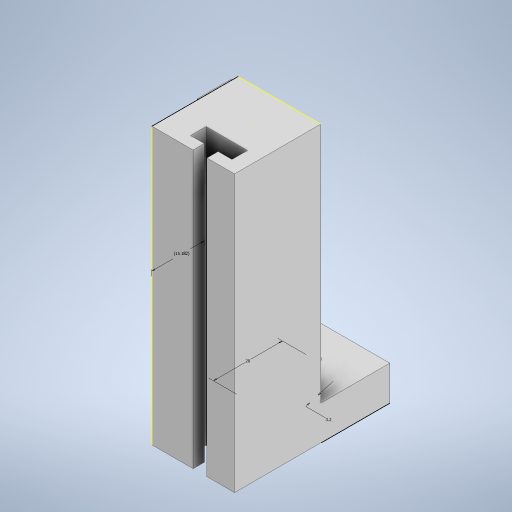
# Autodesk Inventor part: spoutstand
Saved by Autodesk Inventor 2023 (Build 270158000, 158)
## iProperties
Created: 2025-10-02
Part Number: spoutstand
Material: Generic
Document SubType Name: Modeling
Designer: ptato_qo49uko
Density: 1 g/cm^3
Appearance: Default
Author: ptato_qo49uko
Autodesk Inventor part; units mm, degrees
ref_plane "YZ Plane" through (0, 0, 0) normal (1, 0, 0) x (0, 1, 0)
ref_plane "XZ Plane" through (0, 0, 0) normal (0, 1, 0) x (-1, 0, 0)
ref_plane "XY Plane" through (0, 0, 0) normal (0, 0, 1) x (1, 0, 0)
sketch "Sketch1" plane through (0, 0, 0) normal (0, 1, 0) x (-1, 0, 0)
  line L0 (14, 15.1822) -> (-10, 15.1822)
  line L1 (-10, 15.1822) -> (-10, -9.8178)
  line L2 (-10, -9.8178) -> (14, -9.8178)
  line L3 (14, -9.8178) -> (14, 15.1822)
  point P0 (0, 0)
  dimension "d0" = 24
  dimension "d1" = 25
  constraints: 8 end point, 2 parallel, 1 horizontal, 1 perpendicular
  measures "d0" distance of L2.end L1.end
  measures "d1" distance of L1.end L0.end
extrude "Extrusion1" add sketch "Sketch1" along normal blind 80
sketch "Sketch2" plane through (0, 80, 0) normal (0, 1, 0) x (1, 0, 0)
  line L0 (-6, -11.9322) -> (-2, -11.9322)
  line L1 (-2, -11.9322) -> (-2, -15.1822)
  line L2 (2, -15.1822) -> (2, -11.9322)
  line L3 (-2, -15.1822) -> (2, -15.1822)
  line L4 (2, -11.9322) -> (6, -11.9322)
  line L5 (6, -11.9322) -> (6, -7.4322)
  line L6 (-6, -11.9322) -> (-6, -7.4322)
  line L7 (-6, -7.4322) -> (6, -7.4322)
  point P0 (0, 0)
  dimension "d8" = 4
  dimension "d118" = 3.25
  dimension "d119" = 4
  dimension "d120" = 12
  dimension "d121" = 4.5
  dimension "d122" = 4
  constraints: 16 end point, 2 horizontal, 2 vertical, 1 perpendicular, 1 point on line
  measures "d8" distance of L0.start L0.end
  measures "d118" distance of L0.end L1.end
  measures "d119" distance of L2.end L4.end
  measures "d120" distance of L6.end L5.end
  measures "d121" distance of L4.end L5.end
  measures "d122" distance of L1.end L2.start
extrude "Extrusion2" cut sketch "Sketch2" against normal blind 80
sketch "Sketch3" plane through (0, 0, 0) normal (0, -1, 0) x (1, 0, 0)
  line L0 (-14, -9.8178) -> (-14, 15.1822) projected
  line L1 (-14, -9.8178) -> (-14, -29.8178)
  line L2 (-14, -29.8178) -> (10, -29.8178)
  line L3 (10, -9.8178) -> (-14, -9.8178) projected
  line L4 (10, -29.8178) -> (10, -9.8178)
  line L5 (-14, -19.8178) -> (-2, -19.8178)
  circle A0 centre (-2, -19.8178) radius 1.6
  point P0 (0, 0)
  dimension "d121" = 4.5
  dimension "d13" = 20
  dimension "d127" = 3.2
  constraints: 8 end point, 2 perpendicular, 1 centre point, 1 coincident, 1 horizontal, 1 midpoint, 1 vertical
  measures "d13" distance of L0.start L1.end
  measures "d127" diameter of A0
extrude "Extrusion3" add sketch "Sketch3" against normal blind 10 contours A0 | L3 L4 L2 L1
sketch "Sketch4" plane through (-14, 0, 15.1822) normal (-1, 0, 0) x (0, 0, 1)
  line L0 (-25, 2.2028) -> (-15.1822, 2.2028)
  line L1 (-15.1822, 2.2028) -> (-15.1822, 1.2028)
  line L2 (-15.1822, 1.2028) -> (-25, 1.2028)
  line L3 (-25, 1.2028) -> (-25, 2.2028)
  line L4 (-25, 3.2028) -> (-25, 4.2028)
  line L5 (-25, 5.2028) -> (-25, 6.2028)
  line L6 (-25, 7.2028) -> (-25, 8.2028)
  line L7 (-25, 9.2028) -> (-25, 10.2028)
  line L8 (-25, 3.2028) -> (-25, 4.2028)
  line L9 (-25, 6.2028) -> (-15.1822, 6.2028)
  line L10 (-15.1822, 6.2028) -> (-15.1822, 5.2028)
  line L11 (-15.1822, 5.2028) -> (-25, 5.2028)
  line L12 (-25, 5.2028) -> (-25, 6.2028)
  line L13 (-25, 7.2028) -> (-25, 8.2028)
  line L14 (-25, 10.2028) -> (-15.1822, 10.2028)
  line L15 (-15.1822, 10.2028) -> (-15.1822, 9.2028)
  line L16 (-15.1822, 9.2028) -> (-25, 9.2028)
  line L17 (-25, 9.2028) -> (-25, 10.2028)
  line L18 (-25, 11.2036) -> (-25, 12.2036)
  line L19 (-25, 13.2036) -> (-25, 14.2036)
  line L20 (-25, 15.2036) -> (-25, 16.2036)
  line L21 (-25, 11.2036) -> (-25, 12.2036)
  line L22 (-25, 14.2036) -> (-15.1822, 14.2036)
  line L23 (-15.1822, 14.2036) -> (-15.1822, 13.2036)
  line L24 (-15.1822, 13.2036) -> (-25, 13.2036)
  line L25 (-25, 13.2036) -> (-25, 14.2036)
  line L26 (-25, 15.2036) -> (-25, 16.2036)
  line L27 (-15.1822, 18.2036) -> (-15.1822, 17.2036)
  line L28 (-15.1822, 22.2036) -> (-15.1822, 21.2036)
  line L29 (-25, 18.2036) -> (-15.1822, 18.2036)
  line L30 (-15.1822, 17.2036) -> (-25, 17.2036)
  line L31 (-15.1822, 21.2036) -> (-24.9999, 21.2036)
  line L32 (-24.9999, 22.2036) -> (-15.1822, 22.2036)
  line L33 (-25, 17.2036) -> (-25, 18.2036)
  line L34 (-24.9999, 19.2036) -> (-24.9999, 20.2036)
  line L35 (-25, 17.2036) -> (-25, 18.2036)
  line L36 (-24.9999, 19.2036) -> (-24.9999, 20.2036)
  line L37 (-24.9999, 21.2036) -> (-24.9999, 22.2036)
  line L38 (-24.9999, 21.2036) -> (-24.9999, 22.2036)
  line L39 (-24.9999, 23.2036) -> (-24.9999, 24.2036)
  line L40 (-24.9999, 23.2036) -> (-24.9999, 24.2036)
  line L41 (-24.9999, 24.2036) -> (-25, 25.2036)
  line L42 (-25, 10) -> (-25, 80) projected
  line L43 (-25, 25.2036) -> (-15.1821, 25.2036)
  line L44 (-15.1821, 25.2036) -> (-15.1821, 26.2036)
  line L45 (-15.1821, 26.2036) -> (-25, 26.2036)
  line L46 (-25, 26.2036) -> (-25, 25.2036)
  line L47 (-25, 26.2036) -> (-25, 27.2036)
  line L48 (-25, 28.2036) -> (-25, 27.2036)
  line L49 (-25, 28.2036) -> (-25, 29.2036)
  line L50 (-25, 29.2036) -> (-15.1821, 29.2036)
  line L51 (-15.1821, 29.2036) -> (-15.1821, 30.2036)
  line L52 (-15.1821, 30.2036) -> (-25, 30.2036)
  line L53 (-25, 30.2036) -> (-25, 29.2036)
  line L54 (-25, 30.2036) -> (-25, 31.2036)
  line L55 (-25, 32.2036) -> (-25, 31.2036)
  line L56 (-25, 32.2036) -> (-25, 33.2036)
  line L57 (-25, 33.2036) -> (-15.1821, 33.2036)
  line L58 (-15.1821, 33.2036) -> (-15.1821, 34.2036)
  line L59 (-15.1821, 34.2036) -> (-25, 34.2036)
  line L60 (-25, 34.2036) -> (-25, 33.2036)
  line L61 (-25, 34.2036) -> (-25, 35.2036)
  line L62 (-25, 36.2036) -> (-25, 35.2036)
  line L63 (-25, 36.2036) -> (-25, 37.2036)
  line L64 (-25, 37.2036) -> (-15.1821, 37.2036)
  line L65 (-15.1821, 37.2036) -> (-15.1821, 38.2036)
  line L66 (-15.1821, 38.2036) -> (-25, 38.2036)
  line L67 (-25, 38.2036) -> (-25, 37.2036)
  line L68 (-25, 40.2036) -> (-25, 39.2036)
  line L69 (-25, 40.2036) -> (-25, 41.2036)
  line L70 (-25, 41.2036) -> (-15.1822, 41.2036)
  line L71 (-15.1822, 41.2036) -> (-15.1822, 42.2036)
  line L72 (-15.1822, 42.2036) -> (-25, 42.2036)
  line L73 (-25, 42.2036) -> (-25, 41.2036)
  line L74 (-25, 42.2036) -> (-25, 43.2036)
  line L75 (-25, 44.2036) -> (-25, 43.2036)
  line L76 (-25, 44.2036) -> (-25, 45.2036)
  line L77 (-25, 45.2036) -> (-15.1822, 45.2036)
  line L78 (-15.1822, 45.2036) -> (-15.1822, 46.2036)
  line L79 (-15.1822, 46.2036) -> (-25, 46.2036)
  line L80 (-25, 46.2036) -> (-25, 45.2036)
  line L81 (-25, 46.2036) -> (-25, 47.2036)
  line L82 (-25, 48.2036) -> (-25, 47.2036)
  line L83 (-25, 48.2036) -> (-25, 49.2036)
  line L84 (-25, 49.2036) -> (-15.1822, 49.2036)
  line L85 (-15.1822, 49.2036) -> (-15.1822, 50.2036)
  line L86 (-15.1822, 50.2036) -> (-25, 50.2036)
  line L87 (-25, 50.2036) -> (-25, 49.2036)
  line L88 (-25, 50.2036) -> (-25, 51.2036)
  line L89 (-25, 52.2036) -> (-25, 51.2036)
  line L90 (-25, 38.2036) -> (-25, 39.2036)
  line L91 (-15.1821, 57.2036) -> (-15.1821, 58.2036)
  line L92 (-15.1821, 61.2036) -> (-15.1821, 62.2036)
  line L93 (-15.1821, 62.2036) -> (-25, 62.2036)
  line L94 (-25, 61.2036) -> (-15.1821, 61.2036)
  line L95 (-15.1821, 58.2036) -> (-25, 58.2036)
  line L96 (-25, 57.2036) -> (-15.1821, 57.2036)
  line L97 (-25, 53.2036) -> (-15.1821, 53.2036)
  line L98 (-15.1821, 54.2036) -> (-25, 54.2036)
  line L99 (-25, 65.2036) -> (-15.1821, 65.2036)
  line L100 (-15.1821, 66.2036) -> (-25, 66.2036)
  line L101 (-15.1821, 65.2036) -> (-15.1821, 66.2036)
  line L102 (-15.1821, 53.2036) -> (-15.1821, 54.2036)
  line L103 (-25, 54.2036) -> (-25, 53.2036)
  line L104 (-25, 54.2036) -> (-25, 55.2036)
  line L105 (-25, 56.2036) -> (-25, 55.2036)
  line L106 (-25, 56.2036) -> (-25, 57.2036)
  line L107 (-25, 58.2036) -> (-25, 57.2036)
  line L108 (-25, 58.2036) -> (-25, 59.2036)
  line L109 (-25, 66.2036) -> (-25, 65.2036)
  line L110 (-25, 64.2036) -> (-25, 65.2036)
  line L111 (-25, 64.2036) -> (-25, 63.2036)
  line L112 (-25, 62.2036) -> (-25, 63.2036)
  line L113 (-25, 60.2036) -> (-25, 61.2036)
  line L114 (-25, 60.2036) -> (-25, 59.2036)
  line L115 (-25, 62.2036) -> (-25, 61.2036)
  line L116 (-25, 52.2036) -> (-25, 53.2036)
  line L117 (-15.1812, 73.2624) -> (-15.1812, 74.2624)
  line L118 (-15.1812, 69.2624) -> (-15.1812, 70.2624)
  line L119 (-24.9991, 77.2624) -> (-15.1812, 77.2624)
  line L120 (-15.1812, 74.2624) -> (-24.9991, 74.2624)
  line L121 (-24.9991, 73.2624) -> (-15.1812, 73.2624)
  line L122 (-15.1812, 70.2624) -> (-24.9991, 70.2624)
  line L123 (-24.9991, 69.2624) -> (-15.1812, 69.2624)
  line L124 (-15.1812, 78.2624) -> (-24.9991, 78.2624)
  line L125 (-15.1812, 77.2624) -> (-15.1812, 78.2624)
  line L126 (-24.9991, 68.2624) -> (-24.9991, 66.2031)
  line L127 (-24.9991, 70.2624) -> (-24.9991, 69.2624)
  line L128 (-24.9991, 70.2624) -> (-24.9991, 71.2624)
  line L129 (-24.9991, 72.2624) -> (-24.9991, 71.2624)
  line L130 (-24.9991, 72.2624) -> (-24.9991, 73.2624)
  line L131 (-24.9991, 78.2624) -> (-24.9991, 77.2624)
  line L132 (-24.9991, 76.2624) -> (-24.9991, 77.2624)
  line L133 (-24.9991, 74.2624) -> (-24.9991, 75.2624)
  line L134 (-24.9991, 74.2624) -> (-24.9991, 73.2624)
  line L135 (-24.9991, 76.2624) -> (-24.9991, 75.2624)
  line L136 (-25, 66.2036) -> (-25, 67.2036)
  line L137 (-25, 10) -> (-25, 80) projected
  line L138 (-25, 17.2036) -> (-25, 16.2036)
  line L139 (-24.9991, 68.2624) -> (-24.9991, 69.2624)
  line L140 (-25, 4.2028) -> (-15.1812, 4.2028)
  line L141 (-15.1812, 4.2028) -> (-15.1812, 3.2028)
  line L142 (-15.1812, 3.2028) -> (-25, 3.2028)
  line L143 (-25, 3.2028) -> (-25, 4.2028)
  line L144 (-25, 8.2028) -> (-15.1812, 8.2028)
  line L145 (-15.1812, 8.2028) -> (-15.1812, 7.2028)
  line L146 (-15.1812, 7.2028) -> (-25, 7.2028)
  line L147 (-25, 7.2028) -> (-25, 8.2028)
  line L148 (-25, 12.2036) -> (-15.1812, 12.2036)
  line L149 (-15.1812, 12.2036) -> (-15.1812, 11.2036)
  line L150 (-15.1812, 11.2036) -> (-25, 11.2036)
  line L151 (-25, 11.2036) -> (-25, 12.2036)
  line L152 (-25, 16.2036) -> (-15.1812, 16.2036)
  line L153 (-15.1812, 16.2036) -> (-15.1812, 15.2036)
  line L154 (-15.1812, 15.2036) -> (-25, 15.2036)
  line L155 (-25, 15.2036) -> (-25, 16.2036)
  line L156 (-24.9999, 20.2036) -> (-15.1812, 20.2036)
  line L157 (-15.1812, 20.2036) -> (-15.1812, 19.2036)
  line L158 (-15.1812, 19.2036) -> (-24.9999, 19.2036)
  line L159 (-24.9999, 19.2036) -> (-24.9999, 20.2036)
  line L160 (-24.9999, 24.2036) -> (-15.1812, 24.2036)
  line L161 (-15.1812, 24.2036) -> (-15.1812, 23.2036)
  line L162 (-15.1812, 23.2036) -> (-24.9999, 23.2036)
  line L163 (-24.9999, 23.2036) -> (-24.9999, 24.2036)
  line L164 (-25, 28.2036) -> (-15.2728, 28.2036)
  line L165 (-15.2728, 28.2036) -> (-15.2728, 27.2036)
  line L166 (-15.2728, 27.2036) -> (-25, 27.2036)
  line L167 (-25, 27.2036) -> (-25, 28.2036)
  line L168 (-25, 32.2036) -> (-15.1812, 32.2036)
  line L169 (-15.1812, 32.2036) -> (-15.1812, 31.2036)
  line L170 (-15.1812, 31.2036) -> (-25, 31.2036)
  line L171 (-25, 31.2036) -> (-25, 32.2036)
  line L172 (-25, 36.2036) -> (-15.1812, 36.2036)
  line L173 (-15.1812, 36.2036) -> (-15.1812, 35.2036)
  line L174 (-15.1812, 35.2036) -> (-25, 35.2036)
  line L175 (-25, 35.2036) -> (-25, 36.2036)
  line L176 (-25, 40.2036) -> (-15.1812, 40.2036)
  line L177 (-15.1812, 40.2036) -> (-15.1812, 39.2036)
  line L178 (-15.1812, 39.2036) -> (-25, 39.2036)
  line L179 (-25, 39.2036) -> (-25, 40.2036)
  line L180 (-25, 44.2036) -> (-15.1812, 44.2036)
  line L181 (-15.1812, 44.2036) -> (-15.1812, 43.2036)
  line L182 (-15.1812, 43.2036) -> (-25, 43.2036)
  line L183 (-25, 43.2036) -> (-25, 44.2036)
  line L184 (-25, 48.2036) -> (-15.1812, 48.2036)
  line L185 (-15.1812, 48.2036) -> (-15.1812, 47.2036)
  line L186 (-15.1812, 47.2036) -> (-25, 47.2036)
  line L187 (-25, 47.2036) -> (-25, 48.2036)
  line L188 (-25, 52.2036) -> (-15.1812, 52.2036)
  line L189 (-15.1812, 52.2036) -> (-15.1812, 51.2036)
  line L190 (-15.1812, 51.2036) -> (-25, 51.2036)
  line L191 (-25, 51.2036) -> (-25, 52.2036)
  line L192 (-25, 56.2036) -> (-15.1812, 56.2036)
  line L193 (-15.1812, 56.2036) -> (-15.1812, 55.2036)
  line L194 (-15.1812, 55.2036) -> (-25, 55.2036)
  line L195 (-25, 55.2036) -> (-25, 56.2036)
  line L196 (-25, 60.2036) -> (-15.1812, 60.2036)
  line L197 (-15.1812, 60.2036) -> (-15.1812, 59.2036)
  line L198 (-15.1812, 59.2036) -> (-25, 59.2036)
  line L199 (-25, 59.2036) -> (-25, 60.2036)
  line L200 (-25, 64.2036) -> (-15.1812, 64.2036)
  line L201 (-15.1812, 64.2036) -> (-15.1812, 63.2036)
  line L202 (-15.1812, 63.2036) -> (-25, 63.2036)
  line L203 (-25, 63.2036) -> (-25, 64.2036)
  line L204 (-24.9991, 68.2624) -> (-15.1812, 68.2624)
  line L205 (-15.1812, 68.2624) -> (-15.1812, 67.2624)
  line L206 (-15.1812, 67.2624) -> (-24.9991, 67.2624)
  line L207 (-24.9991, 67.2624) -> (-24.9991, 68.2624)
  line L208 (-24.9991, 72.2624) -> (-15.1812, 72.2624)
  line L209 (-15.1812, 72.2624) -> (-15.1812, 71.2624)
  line L210 (-15.1812, 71.2624) -> (-24.9991, 71.2624)
  line L211 (-24.9991, 71.2624) -> (-24.9991, 72.2624)
  line L212 (-24.9991, 76.2624) -> (-15.1812, 76.2624)
  line L213 (-15.1812, 76.2624) -> (-15.1812, 75.2624)
  line L214 (-15.1812, 75.2624) -> (-24.9991, 75.2624)
  line L215 (-24.9991, 75.2624) -> (-24.9991, 76.2624)
  line L216 (-24.9991, 78.2624) -> (-23.9991, 78.2624) construction
  point P0 (-15.1822, 0)
  point P1 (-24, 12.2027)
  point P2 (-20, 17.2036)
  point P3 (-25, 42.2036)
  point P4 (-25, 41.2036)
  point P5 (-25, 46.2036)
  point P6 (-25, 45.2036)
  point P7 (-25, 50.2036)
  point P8 (-25, 49.2036)
  point P9 (-20, 54.2036)
  point P10 (-20, 53.2036)
  point P11 (-20, 58.2036)
  point P12 (-20, 57.2036)
  point P13 (-20, 62.2036)
  point P14 (-20, 61.2036)
  point P15 (-20, 66.2036)
  point P16 (-20, 65.2036)
  point P17 (-20, 70.2037)
  point P18 (-20, 69.2037)
  point P19 (-20, 74.2037)
  point P20 (-20, 73.2037)
  point P21 (-20, 78.2037)
  point P22 (-20, 77.2037)
  point P23 (-25, 16.2036)
  point P24 (-25, 40.2036)
  point P25 (-25, 44.2036)
  point P26 (-25, 43.2036)
  point P27 (-25, 52.2036)
  point P28 (-25, 51.2036)
  dimension "d27" = 1
  dimension "d28" = 1
  dimension "d29" = 1
  dimension "d30" = 1
  dimension "d31" = 1
  dimension "d32" = 1
  dimension "d33" = 1
  dimension "d36" = 1
  dimension "d37" = 1
  dimension "d38" = 1
  dimension "d39" = 1
  dimension "d40" = 1
  dimension "d50" = 1
  dimension "d51" = 1
  dimension "d52" = 1
  dimension "d53" = 1
  dimension "d54" = 1
  dimension "d55" = 1
  dimension "d56" = 1
  dimension "d59" = 1
  dimension "d60" = 1
  dimension "d61" = 1
  dimension "d63" = 1
  dimension "d64" = 1
  dimension "d65" = 1
  dimension "d67" = 1
  dimension "d68" = 1
  dimension "d69" = 1
  dimension "d71" = 1
  dimension "d72" = 1
  dimension "d74" = 1
  dimension "d75" = 1
  dimension "d76" = 1
  dimension "d78" = 1
  dimension "d79" = 1
  dimension "d80" = 1
  dimension "d82" = 1
  dimension "d83" = 1
  dimension "d84" = 1
  dimension "d86" = 1
  dimension "d87" = 1
  dimension "d88" = 1
  dimension "d90" = 1
  dimension "d91" = 1
  dimension "d92" = 1
  dimension "d94" = 1
  dimension "d95" = 1
  dimension "d96" = 1
  dimension "d98" = 1
  dimension "d99" = 1
  dimension "d100" = 1
  dimension "d102" = 1
  dimension "d103" = 1
  dimension "d104" = 1
  dimension "d106" = 1
  dimension "d107" = 1
  dimension "d108" = 1
  dimension "d110" = 1
  dimension "d111" = 1
  dimension "d114" = 1
  dimension "d115" = 1
  dimension "d124" = 1
  constraints: 430 end point, 78 parallel, 40 horizontal, 39 perpendicular, 22 point on line, 1 vertical, 13 other
  measures "d27" distance of L4.start L4.end
  measures "d28" distance of L4.end L5.start
  measures "d29" distance of L5.start L5.end
  measures "d30" distance of L5.end L6.start
  measures "d31" distance of L6.start L6.end
  measures "d32" distance of L6.end L7.start
  measures "d33" distance of L7.start L7.end
  measures "d36" distance of L18.start L18.end
  measures "d37" distance of L18.end L19.start
  measures "d38" distance of L19.start L22.start
  measures "d39" distance of L22.start L20.start
  measures "d40" distance of L20.start L20.end
  measures "d50" distance of L33.start L29.start
  measures "d51" distance of L29.start L34.start
  measures "d52" distance of L34.start L36.end
  measures "d53" distance of L36.end L37.start
  measures "d54" distance of L37.start L32.start
  measures "d55" distance of L32.start L40.start
  measures "d56" distance of L40.start L39.end
  measures "d59" distance of L39.end L41.end
  measures "d60" distance of L44.end L43.end
  measures "d61" distance of L45.end L47.end
  measures "d63" distance of L48.start L49.end
  measures "d64" distance of L51.end L50.end
  measures "d65" distance of L52.end L54.end
  measures "d67" distance of L55.start L56.end
  measures "d68" distance of L58.end L57.end
  measures "d69" distance of L59.end L61.end
  measures "d71" distance of L62.start L63.end
  measures "d72" distance of L65.end L64.end
  measures "d74" distance of L68.start L70.start
  measures "d75" distance of L71.end L71.start
  measures "d76" distance of L72.end L74.end
  measures "d78" distance of L75.start L77.start
  measures "d79" distance of L78.end L78.start
  measures "d80" distance of L79.end L81.end
  measures "d82" distance of L83.start L84.start
  measures "d83" distance of L86.start L84.end
  measures "d84" distance of L86.end L89.end
  measures "d86" distance of L66.end L90.end
  measures "d87" distance of L102.end L102.start
  measures "d88" distance of L103.start L104.end
  measures "d90" distance of L105.start L106.end
  measures "d91" distance of L91.end L96.end
  measures "d92" distance of L95.end L108.end
  measures "d94" distance of L114.start L115.end
  measures "d95" distance of L92.end L92.start
  measures "d96" distance of L115.start L112.end
  measures "d98" distance of L111.start L99.start
  measures "d99" distance of L100.start L99.end
  measures "d100" distance of L89.start L116.end
  measures "d102" distance of L126.start L127.end
  measures "d103" distance of L118.end L118.start
  measures "d104" distance of L127.start L128.end
  measures "d106" distance of L129.start L121.start
  measures "d107" distance of L117.end L117.start
  measures "d108" distance of L120.end L135.end
  measures "d110" distance of L135.start L119.start
  measures "d111" distance of L124.start L119.end
  measures "d114" distance of L100.end L136.end
  measures "d115" distance of L33.start L138.end
  measures "d124" distance of L204.end L205.end
extrude "Extrusion4" add sketch "Sketch4" along normal blind 2
sketch "Sketch5" plane through (-14, 0, 15.1822) normal (-1, 0, 0) x (0, 0, 1)
  line L0 (-15.1822, 41.2036) -> (-15.1822, 42.2036) projected
  line L1 (-15.1822, 42.2036) -> (0, 42.2036)
  line L2 (0, 0) -> (0, 80) projected
  point P0 (-15.1822, 0)
  dimension "d123" = 15.1822
  constraints: 2 end point, 1 horizontal, 1 point on line
  measures "d123" distance of L0.end L1.end
sketch "Sketch6" plane through (0, 80, 0) normal (0, 1, 0) x (1, 0, 0)
  line L0 (10, 9.8178) -> (-14, 9.8178) projected
  line L1 (-14, 9.8178) -> (-14, -15.1822) projected
  line L2 (-14, 9.8178) -> (-14, -15.1822)
  point P0 (0, 0)
  constraints: 2 end point, 1 collinear
extrude "Extrusion5" cut sketch "Sketch3" against normal blind 23.75 contours A0
body "Solid1"
